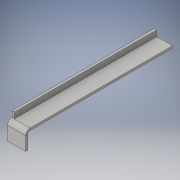
# Autodesk Inventor part: Bent L
Saved by Autodesk Inventor 2016 SP2 (Build 200236200, 236)
## iProperties
Created: 2018-02-01
Part Number: Bent L
Material: Generic
Document SubType Name: Sheet Metal
Designer: CAD
Density: 1 g/cm^3
Sheet Metal Rule: Default
Appearance: Default
Author: CAD
Autodesk Inventor part; units mm, degrees
ref_plane "YZ Plane" through (0, 0, 0) normal (1, 0, 0) x (0, 1, 0)
ref_plane "XZ Plane" through (0, 0, 0) normal (0, 1, 0) x (-1, 0, 0)
ref_plane "XY Plane" through (0, 0, 0) normal (0, 0, 1) x (1, 0, 0)
sketch "Sketch1" plane through (0, 0, 0) normal (0, 0, 1) x (1, 0, 0)
  line L0 (0, 0) -> (25.4, 0)
  line L1 (0, 0) -> (0, 11.43)
  line L2 (3.175, 11.43) -> (3.175, 3.175)
  line L3 (3.175, 3.175) -> (25.4, 3.175)
  line L4 (0, 11.43) -> (3.175, 11.43)
  line L5 (25.4, 3.175) -> (25.4, 0)
  dimension "d0" = 25.4
  dimension "d2" = 11.43
  dimension "d3" = 90
  dimension "d4" = 3.175
  constraints: 12 end point, 2 perpendicular, 1 horizontal, 1 other
  measures "d0" distance of L0.start L0.end
  measures "d2" distance of L0.start L1.end
  measures "d3" angle of L0 L1
  measures "d4" distance between parallel lines of L1 L2
extrude "Extrusion1" add sketch "Sketch1" along normal blind 200.025
sketch "Sketch2" plane through (0, -3.175, 203.2) normal (0, 0, 1) x (1, 0, 0)
  line L0 (25.4, 0) -> (0, 0)
  line L1 (0, 0) -> (0, -19.05)
  line L2 (0, -19.05) -> (25.4, -19.05)
  line L3 (25.4, -19.05) -> (25.4, 0)
  constraints: 6 end point, 1 horizontal, 1 perpendicular, 1 vertical
edge flange "Flange1" height 25.4 angle 90 thickness 3.175 bend radius 3.175 thickness toward (0, 0, 1) relief straight relief width 3.175 relief depth 1.5875 edges at (12.7, 0, 200.025) wall of the first edge with corners at (25.4, -3.175, 203.2) (0, -3.175, 203.2) (0, -22.225, 203.2) (25.4, -22.225, 203.2)
bend "Bend1"
corner "Corner1"
equation "\"d7\" = BendReliefWidth"
equation "\"d8\" = BendReliefDepth"
equation "\"d9\" = MinimumRemnant"
equation "\"d10\" = BendRadius"
equation "\"d13\" = BendRadius"
equation "\"d14\" = CornerReliefSize"
equation "\"d15\" = GapSize"
equation "\"d16\" = JacobiRadiusSize"
equation "\"BendRadius\" = Thickness"
equation "\"BendReliefWidth\" = Thickness"
equation "\"BendReliefDepth\" = 0.5 * Thickness"
equation "\"CornerReliefSize\" = 4 * Thickness"
equation "\"MinimumRemnant\" = 2 * Thickness"
equation "\"TransitionRadius\" = BendRadius"
equation "\"JacobiRadiusSize\" = Thickness"
equation "\"GapSize\" = Thickness"
equation "\"Thickness\" = 3.175"
body "Solid1"
